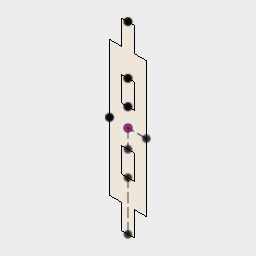
Parametric_object v1 (Autodesk Fusion 360 design; units mm, degrees)
Autodesk Fusion 360 part; units mm, degrees
sketch "Sketch3" plane through (0, 0, 0) normal (0, 0, 1) x (1, 0, 0)
  line L0 (0, 0) -> (0, -3)
  line L1 (0, -3) -> (1.1, -3)
  line L2 (1.1, -3) -> (1.1, -7)
  line L3 (1.1, -7) -> (0, -7)
  line L4 (0, -7) -> (0, -15)
  line L5 (0, -15) -> (1, -15)
  line L6 (1, -15) -> (1, -11)
  line L7 (1, -11) -> (3, -11)
  line L8 (3, -11) -> (3, 0)
  line L9 (3, 0) -> (0, 0)
  line L10 (0, -15) -> (-1, -15)
  line L11 (-1, -15) -> (-1, -11)
  line L12 (-1, -11) -> (-3, -11)
  line L13 (-3, -11) -> (-3, 0)
  line L14 (-1.1, -7) -> (0, -7)
  line L15 (-1.1, -3) -> (-1.1, -7)
  line L16 (0, -3) -> (-1.1, -3)
  line L17 (-3, 11) -> (-3, 0)
  line L18 (-1, 11) -> (-3, 11)
  line L19 (-1, 15) -> (-1, 11)
  line L20 (0, 15) -> (-1, 15)
  line L21 (0, 15) -> (1, 15)
  line L22 (1, 15) -> (1, 11)
  line L23 (1, 11) -> (3, 11)
  line L24 (3, 11) -> (3, 0)
  line L25 (-1.1, 3) -> (-1.1, 7)
  line L26 (0, 3) -> (-1.1, 3)
  line L27 (0, 3) -> (1.1, 3)
  line L28 (1.1, 3) -> (1.1, 7)
  line L29 (1.1, 7) -> (0, 7)
  line L30 (-1.1, 7) -> (0, 7)
  dimension "d35" = 3
  dimension "height" = 2
  dimension "d37" = 1
  dimension "d38" = 1.1
  dimension "d39" = 4
  dimension "d40" = 4
  dimension "d41" = 4
  dimension "d42" = 1.1
  measures "d35" distance of L1 L9
  measures "height" distance of L6.end L7.end
  measures "d37" distance of L4.end L5.end
  measures "d38" distance of L0.end L1.end
  measures "d39" distance of L1.end L2.end
  measures "d40" distance of L3 L7
  measures "d41" distance of L5.end L6.end
  measures "d42" distance of L2.end L3.end
extrude "Extrude3" add sketch "Sketch3" along normal blind 2 contours L0 L1 L2 L3 L4 L5 L6 L7 L8 L9 makes body 1
mirror "Mirror5" about plane through (0, 0, 0) normal (1, 0, 0) of bodies 1 makes body 2
mirror "Mirror6" about plane through (0, 0, 0) normal (0, 1, 0) of bodies 1 2 makes body 3 at (1.3667, 1, 0) makes body 4 at (-1.3667, 1, 0)
extrude "Extrude2" [suppressed]
mirror "Mirror3" [suppressed]
mirror "Mirror4" [suppressed]
chamfer "Chamfer1" [suppressed]
equation "d35 = height * 1.5"
equation "d37 = height / 2"
equation "d38 = height / 2 + 0.1 mm"
equation "d39 = height * 2"
equation "d40 = height * 2"
equation "d41 = height * 2"
equation "d42 = height / 2 + 0.1 mm"
equation "weight = 2 mm"
equation "d47 = weight / 10"
